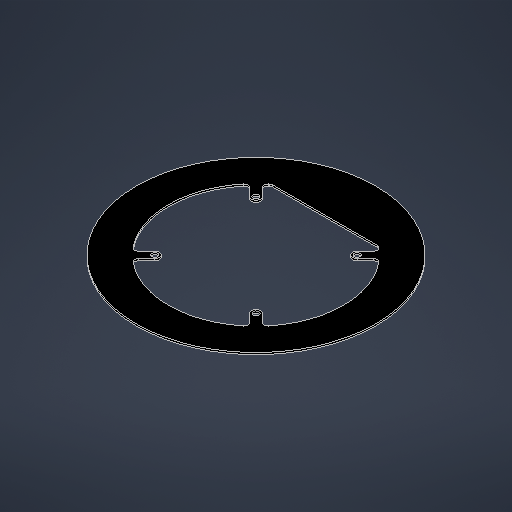
# Autodesk Inventor part: InfraredPCB
Saved by Autodesk Inventor 2025.2 (Build 292293000, 293)
## iProperties
Created: 2023-03-06
Part Number: InfraredPCB
Material: Generic
Document SubType Name: Modeling
Designer: Elias Braun
Density: 1 g/cm^3
Appearance: Default
Author: Elias Braun
Autodesk Inventor part; units mm, degrees
ref_plane "YZ Plane" through (0, 0, 0) normal (1, 0, 0) x (0, 1, 0)
ref_plane "XZ Plane" through (0, 0, 0) normal (0, 1, 0) x (-1, 0, 0)
ref_plane "XY Plane" through (0, 0, 0) normal (0, 0, 1) x (1, 0, 0)
sketch "Sketch3" plane through (0, 0, 0) normal (0, 1, 0) x (-1, 0, 0)
  line L0 (27.5, -27.5) -> (-27.5, -27.5) construction
  line L1 (-27.5, -27.5) -> (-27.5, 27.5) construction
  line L2 (-27.5, 27.5) -> (27.5, 27.5) construction
  line L3 (27.5, 27.5) -> (27.5, -27.5) construction
  line L4 (27.5, -27.5) -> (-27.5, 27.5) construction
  line L5 (-27.5, -27.5) -> (27.5, 27.5) construction
  circle A0 centre (27.5, -27.5) radius 1.6
  circle A1 centre (-27.5, -27.5) radius 1.6
  circle A2 centre (-27.5, 27.5) radius 1.6
  circle A3 centre (27.5, 27.5) radius 1.6
  circle A4 centre (0, 0) radius 65
  line L6 (-27.5, -27.5) -> (-33.5876, -33.5876) construction
  line L7 (-27.5, 27.5) -> (-33.5876, 33.5876) construction
  line L8 (27.5, 27.5) -> (33.5876, 33.5876) construction
  line L9 (27.5, -27.5) -> (33.5876, -33.5876) construction
  line L10 (39.6751, -39.6751) -> (27.5, -27.5) construction
  line L11 (35.3088, -31.7733) -> (29.2678, -25.7322)
  line L12 (25.7322, -29.2678) -> (31.7733, -35.3088)
  arc A5 (29.2678, -25.7322) -> (25.7322, -29.2678) centre (27.5, -27.5) ccw
  line L13 (-39.6751, -39.6751) -> (-27.5, -27.5) construction
  line L14 (-31.7733, -35.3088) -> (-25.7322, -29.2678)
  line L15 (-29.2678, -25.7322) -> (-35.3088, -31.7733)
  arc A6 (-25.7322, -29.2678) -> (-29.2678, -25.7322) centre (-27.5, -27.5) ccw
  line L16 (-39.6751, 39.6751) -> (-27.5, 27.5) construction
  line L17 (-35.3088, 31.7733) -> (-29.2678, 25.7322)
  line L18 (-25.7322, 29.2678) -> (-31.7733, 35.3088)
  arc A7 (-29.2678, 25.7322) -> (-25.7322, 29.2678) centre (-27.5, 27.5) ccw
  line L19 (33.5876, 33.5876) -> (27.5, 27.5) construction
  line L20 (31.7733, 35.3088) -> (25.7322, 29.2678)
  line L21 (29.2678, 25.7322) -> (35.3088, 31.7733)
  arc A8 (25.7322, 29.2678) -> (29.2678, 25.7322) centre (27.5, 27.5) ccw
  arc A9 (31.7733, 35.3088) -> (-31.7733, 35.3088) centre (0, 0) ccw
  arc A10 (-35.3088, 31.7733) -> (-35.3088, -31.7733) centre (0, 0) ccw
  arc A11 (-31.7733, -35.3088) -> (31.7733, -35.3088) centre (0, 0) ccw
  arc A12 (35.3088, -31.7733) -> (35.3088, 31.7733) centre (0, 0) ccw
  line L22 (0, -47.5) -> (0, -37.5) construction
  line L23 (0, -37.5) -> (-29.1548, -37.5)
  line L24 (0, -37.5) -> (29.1548, -37.5)
  dimension "d60" = 55
  dimension "d61" = 55
  dimension "d62" = 3.2
  dimension "d63" = 3.2
  dimension "d64" = 3.2
  dimension "d65" = 3.2
  dimension "d67" = 130
  dimension "d68" = 5
  dimension "d69" = 5
  dimension "d70" = 5
  dimension "d71" = 5
  dimension "d91" = 10
  constraints: 58 end point, 21 point on circle, 13 centre point, 8 tangent, 6 coincident, 6 parallel, 5 midpoint, 4 collinear, 4 point on line, 3 perpendicular, 1 horizontal, 1 vertical
  measures "d60" distance of L0.start L0.end
  measures "d61" distance of L0.end L1.end
  measures "d62" diameter of A0
  measures "d63" diameter of A1
  measures "d64" diameter of A2
  measures "d65" diameter of A3
  measures "d67" diameter of A4
  measures "d68" diameter of A5
  measures "d69" diameter of A6
  measures "d70" diameter of A7
  measures "d71" diameter of A8
  measures "d91" distance of L22.start L22.end
extrude "Extrusion2" add sketch "Sketch3" along normal blind 1 contours A4 | A11 L23 L24
fillet "Fillet1" radius 2 10 edges at (-31.7733, 0.5, 35.3088) (-35.3088, 0.5, 31.7733) (-31.7733, 0.5, -35.3088) (-35.3088, 0.5, -31.7733) (35.3088, 0.5, -31.7733) (31.7733, 0.5, -35.3088) (31.7733, 0.5, 35.3088) (35.3088, 0.5, 31.7733) (-29.1548, 0.5, -37.5) (29.1548, 0.5, -37.5)
sketch "Sketch4" plane through (0, 1, 0) normal (0, 1, 0) x (1, 0, 0)
  circle A0 centre (0, 0) radius 65 projected
  line L0 (0, -65) -> (0, -63) construction
  line L1 (-3, -57) -> (-3, -63)
  line L2 (-3, -63) -> (3, -63)
  line L3 (3, -63) -> (3, -57)
  line L4 (3, -57) -> (-3, -57)
  line L5 (0.8, -52.3) -> (0.8, -55.5)
  line L6 (0.8, -55.5) -> (-0.8, -55.5)
  line L7 (-0.8, -55.5) -> (-0.8, -52.3)
  line L8 (-0.8, -52.3) -> (0.8, -52.3)
  line L9 (1.8, -52.3) -> (1.8, -55.5)
  line L10 (1.8, -55.5) -> (3.4, -55.5)
  line L11 (3.4, -55.5) -> (3.4, -52.3)
  line L12 (3.4, -52.3) -> (1.8, -52.3)
  line L13 (-3.4, -52.3) -> (-3.4, -55.5)
  line L14 (-3.4, -55.5) -> (-1.8, -55.5)
  line L15 (-1.8, -55.5) -> (-1.8, -52.3)
  line L16 (-1.8, -52.3) -> (-3.4, -52.3)
  line L17 (-4.4, -52.3) -> (-4.4, -55.5)
  line L18 (-4.4, -55.5) -> (-6, -55.5)
  line L19 (-6, -55.5) -> (-6, -52.3)
  line L20 (-6, -52.3) -> (-4.4, -52.3)
  line L21 (-4.4, -61.6) -> (-4.4, -58.4)
  line L22 (-4.4, -58.4) -> (-6, -58.4)
  line L23 (-6, -58.4) -> (-6, -61.6)
  line L24 (-6, -61.6) -> (-4.4, -61.6)
  line L25 (18.0977, -52.5764) -> (19.5759, -51.9641)
  line L26 (19.5759, -51.9641) -> (18.3514, -49.0077)
  line L27 (18.3514, -49.0077) -> (16.8732, -49.62)
  line L28 (16.8732, -49.62) -> (18.0977, -52.5764)
  line L29 (15.9493, -50.0027) -> (17.1739, -52.9591)
  line L30 (15.6957, -53.5714) -> (14.4711, -50.615)
  line L31 (14.4711, -50.615) -> (15.9493, -50.0027)
  line L32 (17.1739, -52.9591) -> (15.6957, -53.5714)
  line L33 (18.2836, -55.6384) -> (16.8054, -56.2507)
  line L34 (16.8054, -56.2507) -> (18.03, -59.2071)
  line L35 (18.03, -59.2071) -> (19.5082, -58.5948)
  line L36 (19.5082, -58.5948) -> (18.2836, -55.6384)
  line L37 (19.0413, -53.8092) -> (21.3374, -59.3525)
  line L38 (21.3374, -59.3525) -> (26.8807, -57.0564)
  line L39 (24.8744, -60.0522) -> (24.1091, -58.2044) construction
  line L40 (26.8807, -57.0564) -> (24.5846, -51.5131)
  line L41 (24.5846, -51.5131) -> (19.0413, -53.8092)
  line L42 (20.7534, -48.0128) -> (21.978, -50.9692)
  line L43 (21.978, -50.9692) -> (20.4998, -51.5815)
  line L44 (20.4998, -51.5815) -> (19.2752, -48.625)
  line L45 (19.2752, -48.625) -> (20.7534, -48.0128)
  line L46 (21.6773, -47.6301) -> (22.9019, -50.5865)
  line L47 (22.9019, -50.5865) -> (24.3801, -49.9742)
  line L48 (24.3801, -49.9742) -> (23.1555, -47.0178)
  line L49 (23.1555, -47.0178) -> (21.6773, -47.6301)
  line L50 (36.8403, -41.6486) -> (37.9716, -40.5172)
  line L51 (37.9716, -40.5172) -> (35.7089, -38.2545)
  line L52 (35.7089, -38.2545) -> (34.5775, -39.3858)
  line L53 (34.5775, -39.3858) -> (36.8403, -41.6486)
  line L54 (33.8704, -40.093) -> (36.1332, -42.3557)
  line L55 (35.0018, -43.4871) -> (32.739, -41.2243)
  line L56 (32.739, -41.2243) -> (33.8704, -40.093)
  line L57 (36.1332, -42.3557) -> (35.0018, -43.4871)
  line L58 (38.1838, -44.4063) -> (37.0524, -45.5377)
  line L59 (37.0524, -45.5377) -> (39.3151, -47.8004)
  line L60 (39.3151, -47.8004) -> (40.4465, -46.669)
  line L61 (40.4465, -46.669) -> (38.1838, -44.4063)
  line L62 (38.1838, -42.4264) -> (42.4264, -46.669)
  line L63 (42.4264, -46.669) -> (46.669, -42.4264)
  line L64 (45.9619, -45.9619) -> (44.5477, -44.5477) construction
  line L65 (46.669, -42.4264) -> (42.4264, -38.1838)
  line L66 (42.4264, -38.1838) -> (38.1838, -42.4264)
  line L67 (37.5474, -36.416) -> (39.8101, -38.6787)
  line L68 (39.8101, -38.6787) -> (38.6787, -39.8101)
  line L69 (38.6787, -39.8101) -> (36.416, -37.5474)
  line L70 (36.416, -37.5474) -> (37.5474, -36.416)
  line L71 (38.2545, -35.7089) -> (40.5172, -37.9716)
  line L72 (40.5172, -37.9716) -> (41.6486, -36.8403)
  line L73 (41.6486, -36.8403) -> (39.3858, -34.5775)
  line L74 (39.3858, -34.5775) -> (38.2545, -35.7089)
  line L75 (49.9742, -24.3801) -> (50.5865, -22.9019)
  line L76 (50.5865, -22.9019) -> (47.6301, -21.6773)
  line L77 (47.6301, -21.6773) -> (47.0178, -23.1555)
  line L78 (47.0178, -23.1555) -> (49.9742, -24.3801)
  line L79 (46.6351, -24.0794) -> (49.5915, -25.304)
  line L80 (48.9792, -26.7822) -> (46.0228, -25.5576)
  line L81 (46.0228, -25.5576) -> (46.6351, -24.0794)
  line L82 (49.5915, -25.304) -> (48.9792, -26.7822)
  line L83 (52.2708, -26.4138) -> (51.6585, -27.892)
  line L84 (51.6585, -27.892) -> (54.6149, -29.1166)
  line L85 (54.6149, -29.1166) -> (55.2272, -27.6384)
  line L86 (55.2272, -27.6384) -> (52.2708, -26.4138)
  line L87 (51.5131, -24.5846) -> (57.0564, -26.8807)
  line L88 (57.0564, -26.8807) -> (59.3525, -21.3374)
  line L89 (60.0522, -24.8744) -> (58.2044, -24.1091) construction
  line L90 (59.3525, -21.3374) -> (53.8092, -19.0413)
  line L91 (53.8092, -19.0413) -> (51.5131, -24.5846)
  line L92 (48.625, -19.2752) -> (51.5815, -20.4998)
  line L93 (51.5815, -20.4998) -> (50.9692, -21.978)
  line L94 (50.9692, -21.978) -> (48.0128, -20.7534)
  line L95 (48.0128, -20.7534) -> (48.625, -19.2752)
  line L96 (49.0077, -18.3514) -> (51.9641, -19.5759)
  line L97 (51.9641, -19.5759) -> (52.5764, -18.0977)
  line L98 (52.5764, -18.0977) -> (49.62, -16.8732)
  line L99 (49.62, -16.8732) -> (49.0077, -18.3514)
  line L100 (55.5, -3.4) -> (55.5, -1.8)
  line L101 (55.5, -1.8) -> (52.3, -1.8)
  line L102 (52.3, -1.8) -> (52.3, -3.4)
  line L103 (52.3, -3.4) -> (55.5, -3.4)
  line L104 (52.3, -4.4) -> (55.5, -4.4)
  line L105 (55.5, -6) -> (52.3, -6)
  line L106 (52.3, -6) -> (52.3, -4.4)
  line L107 (55.5, -4.4) -> (55.5, -6)
  line L108 (58.4, -4.4) -> (58.4, -6)
  line L109 (58.4, -6) -> (61.6, -6)
  line L110 (61.6, -6) -> (61.6, -4.4)
  line L111 (61.6, -4.4) -> (58.4, -4.4)
  line L112 (57, -3) -> (63, -3)
  line L113 (63, -3) -> (63, 3)
  line L114 (65, 0) -> (63, 0) construction
  line L115 (63, 3) -> (57, 3)
  line L116 (57, 3) -> (57, -3)
  line L117 (52.3, 0.8) -> (55.5, 0.8)
  line L118 (55.5, 0.8) -> (55.5, -0.8)
  line L119 (55.5, -0.8) -> (52.3, -0.8)
  line L120 (52.3, -0.8) -> (52.3, 0.8)
  line L121 (52.3, 1.8) -> (55.5, 1.8)
  line L122 (55.5, 1.8) -> (55.5, 3.4)
  line L123 (55.5, 3.4) -> (52.3, 3.4)
  line L124 (52.3, 3.4) -> (52.3, 1.8)
  line L125 (52.5764, 18.0977) -> (51.9641, 19.5759)
  line L126 (51.9641, 19.5759) -> (49.0077, 18.3514)
  line L127 (49.0077, 18.3514) -> (49.62, 16.8732)
  line L128 (49.62, 16.8732) -> (52.5764, 18.0977)
  line L129 (50.0027, 15.9493) -> (52.9591, 17.1739)
  line L130 (53.5714, 15.6957) -> (50.615, 14.4711)
  line L131 (50.615, 14.4711) -> (50.0027, 15.9493)
  line L132 (52.9591, 17.1739) -> (53.5714, 15.6957)
  line L133 (55.6384, 18.2836) -> (56.2507, 16.8054)
  line L134 (56.2507, 16.8054) -> (59.2071, 18.03)
  line L135 (59.2071, 18.03) -> (58.5948, 19.5082)
  line L136 (58.5948, 19.5082) -> (55.6384, 18.2836)
  line L137 (53.8092, 19.0413) -> (59.3525, 21.3374)
  line L138 (59.3525, 21.3374) -> (57.0564, 26.8807)
  line L139 (60.0522, 24.8744) -> (58.2044, 24.1091) construction
  line L140 (57.0564, 26.8807) -> (51.5131, 24.5846)
  line L141 (51.5131, 24.5846) -> (53.8092, 19.0413)
  line L142 (48.0128, 20.7534) -> (50.9692, 21.978)
  line L143 (50.9692, 21.978) -> (51.5815, 20.4998)
  line L144 (51.5815, 20.4998) -> (48.625, 19.2752)
  line L145 (48.625, 19.2752) -> (48.0128, 20.7534)
  line L146 (47.6301, 21.6773) -> (50.5865, 22.9019)
  line L147 (50.5865, 22.9019) -> (49.9742, 24.3801)
  line L148 (49.9742, 24.3801) -> (47.0178, 23.1555)
  line L149 (47.0178, 23.1555) -> (47.6301, 21.6773)
  line L150 (41.6486, 36.8403) -> (40.5172, 37.9716)
  line L151 (40.5172, 37.9716) -> (38.2545, 35.7089)
  line L152 (38.2545, 35.7089) -> (39.3858, 34.5775)
  line L153 (39.3858, 34.5775) -> (41.6486, 36.8403)
  line L154 (40.093, 33.8704) -> (42.3557, 36.1332)
  line L155 (43.4871, 35.0018) -> (41.2243, 32.739)
  line L156 (41.2243, 32.739) -> (40.093, 33.8704)
  line L157 (42.3557, 36.1332) -> (43.4871, 35.0018)
  line L158 (44.4063, 38.1838) -> (45.5377, 37.0524)
  line L159 (45.5377, 37.0524) -> (47.8004, 39.3151)
  line L160 (47.8004, 39.3151) -> (46.669, 40.4465)
  line L161 (46.669, 40.4465) -> (44.4063, 38.1838)
  line L162 (42.4264, 38.1838) -> (46.669, 42.4264)
  line L163 (46.669, 42.4264) -> (42.4264, 46.669)
  line L164 (45.9619, 45.9619) -> (44.5477, 44.5477) construction
  line L165 (42.4264, 46.669) -> (38.1838, 42.4264)
  line L166 (38.1838, 42.4264) -> (42.4264, 38.1838)
  line L167 (36.416, 37.5474) -> (38.6787, 39.8101)
  line L168 (38.6787, 39.8101) -> (39.8101, 38.6787)
  line L169 (39.8101, 38.6787) -> (37.5474, 36.416)
  line L170 (37.5474, 36.416) -> (36.416, 37.5474)
  line L171 (35.7089, 38.2545) -> (37.9716, 40.5172)
  line L172 (37.9716, 40.5172) -> (36.8403, 41.6486)
  line L173 (36.8403, 41.6486) -> (34.5775, 39.3858)
  line L174 (34.5775, 39.3858) -> (35.7089, 38.2545)
  line L175 (24.3801, 49.9742) -> (22.9019, 50.5865)
  line L176 (22.9019, 50.5865) -> (21.6773, 47.6301)
  line L177 (21.6773, 47.6301) -> (23.1555, 47.0178)
  line L178 (23.1555, 47.0178) -> (24.3801, 49.9742)
  line L179 (24.0794, 46.6351) -> (25.304, 49.5915)
  line L180 (26.7822, 48.9792) -> (25.5576, 46.0228)
  line L181 (25.5576, 46.0228) -> (24.0794, 46.6351)
  line L182 (25.304, 49.5915) -> (26.7822, 48.9792)
  line L183 (26.4138, 52.2708) -> (27.892, 51.6585)
  line L184 (27.892, 51.6585) -> (29.1166, 54.6149)
  line L185 (29.1166, 54.6149) -> (27.6384, 55.2272)
  line L186 (27.6384, 55.2272) -> (26.4138, 52.2708)
  line L187 (24.5846, 51.5131) -> (26.8807, 57.0564)
  line L188 (26.8807, 57.0564) -> (21.3374, 59.3525)
  line L189 (24.8744, 60.0522) -> (24.1091, 58.2044) construction
  line L190 (21.3374, 59.3525) -> (19.0413, 53.8092)
  line L191 (19.0413, 53.8092) -> (24.5846, 51.5131)
  line L192 (19.2752, 48.625) -> (20.4998, 51.5815)
  line L193 (20.4998, 51.5815) -> (21.978, 50.9692)
  line L194 (21.978, 50.9692) -> (20.7534, 48.0128)
  line L195 (20.7534, 48.0128) -> (19.2752, 48.625)
  line L196 (18.3514, 49.0077) -> (19.5759, 51.9641)
  line L197 (19.5759, 51.9641) -> (18.0977, 52.5764)
  line L198 (18.0977, 52.5764) -> (16.8732, 49.62)
  line L199 (16.8732, 49.62) -> (18.3514, 49.0077)
  line L200 (3.4, 55.5) -> (1.8, 55.5)
  line L201 (1.8, 55.5) -> (1.8, 52.3)
  line L202 (1.8, 52.3) -> (3.4, 52.3)
  line L203 (3.4, 52.3) -> (3.4, 55.5)
  line L204 (4.4, 52.3) -> (4.4, 55.5)
  line L205 (6, 55.5) -> (6, 52.3)
  line L206 (6, 52.3) -> (4.4, 52.3)
  line L207 (4.4, 55.5) -> (6, 55.5)
  line L208 (4.4, 58.4) -> (6, 58.4)
  line L209 (6, 58.4) -> (6, 61.6)
  line L210 (6, 61.6) -> (4.4, 61.6)
  line L211 (4.4, 61.6) -> (4.4, 58.4)
  line L212 (3, 57) -> (3, 63)
  line L213 (3, 63) -> (-3, 63)
  line L214 (0, 65) -> (0, 63) construction
  line L215 (-3, 63) -> (-3, 57)
  line L216 (-3, 57) -> (3, 57)
  line L217 (-0.8, 52.3) -> (-0.8, 55.5)
  line L218 (-0.8, 55.5) -> (0.8, 55.5)
  line L219 (0.8, 55.5) -> (0.8, 52.3)
  line L220 (0.8, 52.3) -> (-0.8, 52.3)
  line L221 (-1.8, 52.3) -> (-1.8, 55.5)
  line L222 (-1.8, 55.5) -> (-3.4, 55.5)
  line L223 (-3.4, 55.5) -> (-3.4, 52.3)
  line L224 (-3.4, 52.3) -> (-1.8, 52.3)
  line L225 (-18.0977, 52.5764) -> (-19.5759, 51.9641)
  line L226 (-19.5759, 51.9641) -> (-18.3514, 49.0077)
  line L227 (-18.3514, 49.0077) -> (-16.8732, 49.62)
  line L228 (-16.8732, 49.62) -> (-18.0977, 52.5764)
  line L229 (-15.9493, 50.0027) -> (-17.1739, 52.9591)
  line L230 (-15.6957, 53.5714) -> (-14.4711, 50.615)
  line L231 (-14.4711, 50.615) -> (-15.9493, 50.0027)
  line L232 (-17.1739, 52.9591) -> (-15.6957, 53.5714)
  line L233 (-18.2836, 55.6384) -> (-16.8054, 56.2507)
  line L234 (-16.8054, 56.2507) -> (-18.03, 59.2071)
  line L235 (-18.03, 59.2071) -> (-19.5082, 58.5948)
  line L236 (-19.5082, 58.5948) -> (-18.2836, 55.6384)
  line L237 (-19.0413, 53.8092) -> (-21.3374, 59.3525)
  line L238 (-21.3374, 59.3525) -> (-26.8807, 57.0564)
  line L239 (-24.8744, 60.0522) -> (-24.1091, 58.2044) construction
  line L240 (-26.8807, 57.0564) -> (-24.5846, 51.5131)
  line L241 (-24.5846, 51.5131) -> (-19.0413, 53.8092)
  line L242 (-20.7534, 48.0128) -> (-21.978, 50.9692)
  line L243 (-21.978, 50.9692) -> (-20.4998, 51.5815)
  line L244 (-20.4998, 51.5815) -> (-19.2752, 48.625)
  line L245 (-19.2752, 48.625) -> (-20.7534, 48.0128)
  line L246 (-21.6773, 47.6301) -> (-22.9019, 50.5865)
  line L247 (-22.9019, 50.5865) -> (-24.3801, 49.9742)
  line L248 (-24.3801, 49.9742) -> (-23.1555, 47.0178)
  line L249 (-23.1555, 47.0178) -> (-21.6773, 47.6301)
  line L250 (-36.8403, 41.6486) -> (-37.9716, 40.5172)
  line L251 (-37.9716, 40.5172) -> (-35.7089, 38.2545)
  line L252 (-35.7089, 38.2545) -> (-34.5775, 39.3858)
  line L253 (-34.5775, 39.3858) -> (-36.8403, 41.6486)
  line L254 (-33.8704, 40.093) -> (-36.1332, 42.3557)
  line L255 (-35.0018, 43.4871) -> (-32.739, 41.2243)
  line L256 (-32.739, 41.2243) -> (-33.8704, 40.093)
  line L257 (-36.1332, 42.3557) -> (-35.0018, 43.4871)
  line L258 (-38.1838, 44.4063) -> (-37.0524, 45.5377)
  line L259 (-37.0524, 45.5377) -> (-39.3151, 47.8004)
  line L260 (-39.3151, 47.8004) -> (-40.4465, 46.669)
  line L261 (-40.4465, 46.669) -> (-38.1838, 44.4063)
  line L262 (-38.1838, 42.4264) -> (-42.4264, 46.669)
  line L263 (-42.4264, 46.669) -> (-46.669, 42.4264)
  line L264 (-45.9619, 45.9619) -> (-44.5477, 44.5477) construction
  line L265 (-46.669, 42.4264) -> (-42.4264, 38.1838)
  line L266 (-42.4264, 38.1838) -> (-38.1838, 42.4264)
  line L267 (-37.5474, 36.416) -> (-39.8101, 38.6787)
  line L268 (-39.8101, 38.6787) -> (-38.6787, 39.8101)
  line L269 (-38.6787, 39.8101) -> (-36.416, 37.5474)
  line L270 (-36.416, 37.5474) -> (-37.5474, 36.416)
  line L271 (-38.2545, 35.7089) -> (-40.5172, 37.9716)
  line L272 (-40.5172, 37.9716) -> (-41.6486, 36.8403)
  line L273 (-41.6486, 36.8403) -> (-39.3858, 34.5775)
  line L274 (-39.3858, 34.5775) -> (-38.2545, 35.7089)
  line L275 (-49.9742, 24.3801) -> (-50.5865, 22.9019)
  line L276 (-50.5865, 22.9019) -> (-47.6301, 21.6773)
  line L277 (-47.6301, 21.6773) -> (-47.0178, 23.1555)
  line L278 (-47.0178, 23.1555) -> (-49.9742, 24.3801)
  line L279 (-46.6351, 24.0794) -> (-49.5915, 25.304)
  line L280 (-48.9792, 26.7822) -> (-46.0228, 25.5576)
  line L281 (-46.0228, 25.5576) -> (-46.6351, 24.0794)
  line L282 (-49.5915, 25.304) -> (-48.9792, 26.7822)
  line L283 (-52.2708, 26.4138) -> (-51.6585, 27.892)
  line L284 (-51.6585, 27.892) -> (-54.6149, 29.1166)
  line L285 (-54.6149, 29.1166) -> (-55.2272, 27.6384)
  line L286 (-55.2272, 27.6384) -> (-52.2708, 26.4138)
  line L287 (-51.5131, 24.5846) -> (-57.0564, 26.8807)
  line L288 (-57.0564, 26.8807) -> (-59.3525, 21.3374)
  line L289 (-60.0522, 24.8744) -> (-58.2044, 24.1091) construction
  line L290 (-59.3525, 21.3374) -> (-53.8092, 19.0413)
  line L291 (-53.8092, 19.0413) -> (-51.5131, 24.5846)
  line L292 (-48.625, 19.2752) -> (-51.5815, 20.4998)
  line L293 (-51.5815, 20.4998) -> (-50.9692, 21.978)
  line L294 (-50.9692, 21.978) -> (-48.0128, 20.7534)
  line L295 (-48.0128, 20.7534) -> (-48.625, 19.2752)
  line L296 (-49.0077, 18.3514) -> (-51.9641, 19.5759)
  line L297 (-51.9641, 19.5759) -> (-52.5764, 18.0977)
  line L298 (-52.5764, 18.0977) -> (-49.62, 16.8732)
  line L299 (-49.62, 16.8732) -> (-49.0077, 18.3514)
  line L300 (-55.5, 3.4) -> (-55.5, 1.8)
  line L301 (-55.5, 1.8) -> (-52.3, 1.8)
  line L302 (-52.3, 1.8) -> (-52.3, 3.4)
  line L303 (-52.3, 3.4) -> (-55.5, 3.4)
  line L304 (-52.3, 4.4) -> (-55.5, 4.4)
  line L305 (-55.5, 6) -> (-52.3, 6)
  line L306 (-52.3, 6) -> (-52.3, 4.4)
  line L307 (-55.5, 4.4) -> (-55.5, 6)
  line L308 (-58.4, 4.4) -> (-58.4, 6)
  line L309 (-58.4, 6) -> (-61.6, 6)
  line L310 (-61.6, 6) -> (-61.6, 4.4)
  line L311 (-61.6, 4.4) -> (-58.4, 4.4)
  line L312 (-57, 3) -> (-63, 3)
  line L313 (-63, 3) -> (-63, -3)
  line L314 (-65, 0) -> (-63, 0) construction
  line L315 (-63, -3) -> (-57, -3)
  line L316 (-57, -3) -> (-57, 3)
  line L317 (-52.3, -0.8) -> (-55.5, -0.8)
  line L318 (-55.5, -0.8) -> (-55.5, 0.8)
  line L319 (-55.5, 0.8) -> (-52.3, 0.8)
  line L320 (-52.3, 0.8) -> (-52.3, -0.8)
  line L321 (-52.3, -1.8) -> (-55.5, -1.8)
  line L322 (-55.5, -1.8) -> (-55.5, -3.4)
  line L323 (-55.5, -3.4) -> (-52.3, -3.4)
  line L324 (-52.3, -3.4) -> (-52.3, -1.8)
  line L325 (-52.5764, -18.0977) -> (-51.9641, -19.5759)
  line L326 (-51.9641, -19.5759) -> (-49.0077, -18.3514)
  line L327 (-49.0077, -18.3514) -> (-49.62, -16.8732)
  line L328 (-49.62, -16.8732) -> (-52.5764, -18.0977)
  line L329 (-50.0027, -15.9493) -> (-52.9591, -17.1739)
  line L330 (-53.5714, -15.6957) -> (-50.615, -14.4711)
  line L331 (-50.615, -14.4711) -> (-50.0027, -15.9493)
  line L332 (-52.9591, -17.1739) -> (-53.5714, -15.6957)
  line L333 (-55.6384, -18.2836) -> (-56.2507, -16.8054)
  line L334 (-56.2507, -16.8054) -> (-59.2071, -18.03)
  line L335 (-59.2071, -18.03) -> (-58.5948, -19.5082)
  line L336 (-58.5948, -19.5082) -> (-55.6384, -18.2836)
  line L337 (-53.8092, -19.0413) -> (-59.3525, -21.3374)
  line L338 (-59.3525, -21.3374) -> (-57.0564, -26.8807)
  line L339 (-60.0522, -24.8744) -> (-58.2044, -24.1091) construction
  line L340 (-57.0564, -26.8807) -> (-51.5131, -24.5846)
  line L341 (-51.5131, -24.5846) -> (-53.8092, -19.0413)
  line L342 (-48.0128, -20.7534) -> (-50.9692, -21.978)
  line L343 (-50.9692, -21.978) -> (-51.5815, -20.4998)
  line L344 (-51.5815, -20.4998) -> (-48.625, -19.2752)
  line L345 (-48.625, -19.2752) -> (-48.0128, -20.7534)
  line L346 (-47.6301, -21.6773) -> (-50.5865, -22.9019)
  line L347 (-50.5865, -22.9019) -> (-49.9742, -24.3801)
  line L348 (-49.9742, -24.3801) -> (-47.0178, -23.1555)
  line L349 (-47.0178, -23.1555) -> (-47.6301, -21.6773)
  line L350 (-41.6486, -36.8403) -> (-40.5172, -37.9716)
  line L351 (-40.5172, -37.9716) -> (-38.2545, -35.7089)
  line L352 (-38.2545, -35.7089) -> (-39.3858, -34.5775)
  line L353 (-39.3858, -34.5775) -> (-41.6486, -36.8403)
  line L354 (-40.093, -33.8704) -> (-42.3557, -36.1332)
  line L355 (-43.4871, -35.0018) -> (-41.2243, -32.739)
  line L356 (-41.2243, -32.739) -> (-40.093, -33.8704)
  line L357 (-42.3557, -36.1332) -> (-43.4871, -35.0018)
  line L358 (-44.4063, -38.1838) -> (-45.5377, -37.0524)
  line L359 (-45.5377, -37.0524) -> (-47.8004, -39.3151)
  line L360 (-47.8004, -39.3151) -> (-46.669, -40.4465)
  line L361 (-46.669, -40.4465) -> (-44.4063, -38.1838)
  line L362 (-42.4264, -38.1838) -> (-46.669, -42.4264)
  line L363 (-46.669, -42.4264) -> (-42.4264, -46.669)
  line L364 (-45.9619, -45.9619) -> (-44.5477, -44.5477) construction
  line L365 (-42.4264, -46.669) -> (-38.1838, -42.4264)
  line L366 (-38.1838, -42.4264) -> (-42.4264, -38.1838)
  line L367 (-36.416, -37.5474) -> (-38.6787, -39.8101)
  line L368 (-38.6787, -39.8101) -> (-39.8101, -38.6787)
  line L369 (-39.8101, -38.6787) -> (-37.5474, -36.416)
  line L370 (-37.5474, -36.416) -> (-36.416, -37.5474)
  line L371 (-35.7089, -38.2545) -> (-37.9716, -40.5172)
  line L372 (-37.9716, -40.5172) -> (-36.8403, -41.6486)
  line L373 (-36.8403, -41.6486) -> (-34.5775, -39.3858)
  line L374 (-34.5775, -39.3858) -> (-35.7089, -38.2545)
  line L375 (-24.3801, -49.9742) -> (-22.9019, -50.5865)
  line L376 (-22.9019, -50.5865) -> (-21.6773, -47.6301)
  line L377 (-21.6773, -47.6301) -> (-23.1555, -47.0178)
  line L378 (-23.1555, -47.0178) -> (-24.3801, -49.9742)
  line L379 (-24.0794, -46.6351) -> (-25.304, -49.5915)
  line L380 (-26.7822, -48.9792) -> (-25.5576, -46.0228)
  line L381 (-25.5576, -46.0228) -> (-24.0794, -46.6351)
  line L382 (-25.304, -49.5915) -> (-26.7822, -48.9792)
  line L383 (-26.4138, -52.2708) -> (-27.892, -51.6585)
  line L384 (-27.892, -51.6585) -> (-29.1166, -54.6149)
  line L385 (-29.1166, -54.6149) -> (-27.6384, -55.2272)
  line L386 (-27.6384, -55.2272) -> (-26.4138, -52.2708)
  line L387 (-24.5846, -51.5131) -> (-26.8807, -57.0564)
  line L388 (-26.8807, -57.0564) -> (-21.3374, -59.3525)
  line L389 (-24.8744, -60.0522) -> (-24.1091, -58.2044) construction
  line L390 (-21.3374, -59.3525) -> (-19.0413, -53.8092)
  line L391 (-19.0413, -53.8092) -> (-24.5846, -51.5131)
  line L392 (-19.2752, -48.625) -> (-20.4998, -51.5815)
  line L393 (-20.4998, -51.5815) -> (-21.978, -50.9692)
  line L394 (-21.978, -50.9692) -> (-20.7534, -48.0128)
  line L395 (-20.7534, -48.0128) -> (-19.2752, -48.625)
  line L396 (-18.3514, -49.0077) -> (-19.5759, -51.9641)
  line L397 (-19.5759, -51.9641) -> (-18.0977, -52.5764)
  line L398 (-18.0977, -52.5764) -> (-16.8732, -49.62)
  line L399 (-16.8732, -49.62) -> (-18.3514, -49.0077)
  point P0 (0, -53.9)
  point P1 (0, -60)
  point P2 (2.6, -53.9)
  point P3 (-2.6, -53.9)
  point P4 (-5.2, -53.9)
  point P5 (-5.2, -60)
  point P6 (18.1568, -57.4227)
  point P7 (15.8225, -51.7871)
  point P8 (18.2246, -50.7921)
  point P9 (23.0287, -48.8021)
  point P10 (22.961, -55.4328)
  point P11 (20.6266, -49.7971)
  point P12 (38.7495, -46.1034)
  point P13 (34.4361, -41.79)
  point P14 (36.2746, -39.9515)
  point P15 (39.9515, -36.2746)
  point P16 (42.4264, -42.4264)
  point P17 (38.1131, -38.1131)
  point P18 (53.4428, -27.7652)
  point P19 (47.8072, -25.4308)
  point P20 (48.8021, -23.0287)
  point P21 (50.7921, -18.2246)
  point P22 (55.4328, -22.961)
  point P23 (49.7971, -20.6266)
  point P24 (60, -5.2)
  point P25 (53.9, -5.2)
  point P26 (53.9, -2.6)
  point P27 (53.9, 2.6)
  point P28 (60, 0)
  point P29 (53.9, 0)
  point P30 (57.4227, 18.1568)
  point P31 (51.7871, 15.8225)
  point P32 (50.7921, 18.2246)
  point P33 (48.8021, 23.0287)
  point P34 (55.4328, 22.961)
  point P35 (49.7971, 20.6266)
  point P36 (46.1034, 38.7495)
  point P37 (41.79, 34.4361)
  point P38 (39.9515, 36.2746)
  point P39 (36.2746, 39.9515)
  point P40 (42.4264, 42.4264)
  point P41 (38.1131, 38.1131)
  point P42 (27.7652, 53.4428)
  point P43 (25.4308, 47.8072)
  point P44 (23.0287, 48.8021)
  point P45 (18.2246, 50.7921)
  point P46 (22.961, 55.4328)
  point P47 (20.6266, 49.7971)
  point P48 (5.2, 60)
  point P49 (5.2, 53.9)
  point P50 (2.6, 53.9)
  point P51 (-2.6, 53.9)
  point P52 (0, 60)
  point P53 (0, 53.9)
  point P54 (-18.1568, 57.4227)
  point P55 (-15.8225, 51.7871)
  point P56 (-18.2246, 50.7921)
  point P57 (-23.0287, 48.8021)
  point P58 (-22.961, 55.4328)
  point P59 (-20.6266, 49.7971)
  point P60 (-38.7495, 46.1034)
  point P61 (-34.4361, 41.79)
  point P62 (-36.2746, 39.9515)
  point P63 (-39.9515, 36.2746)
  point P64 (-42.4264, 42.4264)
  point P65 (-38.1131, 38.1131)
  point P66 (-53.4428, 27.7652)
  point P67 (-47.8072, 25.4308)
  point P68 (-48.8021, 23.0287)
  point P69 (-50.7921, 18.2246)
  point P70 (-55.4328, 22.961)
  point P71 (-49.7971, 20.6266)
  point P72 (-60, 5.2)
  point P73 (-53.9, 5.2)
  point P74 (-53.9, 2.6)
  point P75 (-53.9, -2.6)
  point P76 (-60, 0)
  point P77 (-53.9, 0)
  point P78 (-57.4227, -18.1568)
  point P79 (-51.7871, -15.8225)
  point P80 (-50.7921, -18.2246)
  point P81 (-48.8021, -23.0287)
  point P82 (-55.4328, -22.961)
  point P83 (-49.7971, -20.6266)
  point P84 (-46.1034, -38.7495)
  point P85 (-41.79, -34.4361)
  point P86 (-39.9515, -36.2746)
  point P87 (-36.2746, -39.9515)
  point P88 (-42.4264, -42.4264)
  point P89 (-38.1131, -38.1131)
  point P90 (-27.7652, -53.4428)
  point P91 (-25.4308, -47.8072)
  point P92 (-23.0287, -48.8021)
  point P93 (-18.2246, -50.7921)
  point P94 (-22.961, -55.4328)
  point P95 (-20.6266, -49.7971)
  dimension "d89" = 360
  constraints: 800 end point, 6 parallel, 3 perpendicular, 2 coincident, 2 vertical, 1 vertical alignment, 928 other
sketch "Sketch5" plane through (0, 1, 0) normal (0, 1, 0) x (1, 0, 0)
  circle A0 centre (0, 0) radius 65
  line L0 (0, -65) -> (0, -63) construction
  line L1 (-3, -57) -> (-3, -63)
  line L2 (-3, -63) -> (3, -63)
  line L3 (3, -63) -> (3, -57)
  line L4 (3, -57) -> (-3, -57)
  line L5 (0.8, -52.3) -> (0.8, -55.5)
  line L6 (0.8, -55.5) -> (-0.8, -55.5)
  line L7 (-0.8, -55.5) -> (-0.8, -52.3)
  line L8 (-0.8, -52.3) -> (0.8, -52.3)
  line L9 (1.8, -52.3) -> (1.8, -55.5)
  line L10 (1.8, -55.5) -> (3.4, -55.5)
  line L11 (3.4, -55.5) -> (3.4, -52.3)
  line L12 (3.4, -52.3) -> (1.8, -52.3)
  line L13 (-1.8, -52.3) -> (-3.4, -52.3)
  line L14 (-3.4, -52.3) -> (-3.4, -55.5)
  line L15 (-3.4, -55.5) -> (-1.8, -55.5)
  line L16 (-1.8, -55.5) -> (-1.8, -52.3)
  line L17 (-4.4, -52.3) -> (-4.4, -55.5)
  line L18 (-6, -55.5) -> (-6, -52.3)
  line L19 (-6, -52.3) -> (-4.4, -52.3)
  line L20 (-4.4, -55.5) -> (-6, -55.5)
  line L21 (-4.4, -61.6) -> (-4.4, -58.4)
  line L22 (-4.4, -58.4) -> (-6, -58.4)
  line L23 (-6, -58.4) -> (-6, -61.6)
  line L24 (-6, -61.6) -> (-4.4, -61.6)
  line L25 (18.0977, -52.5764) -> (19.5759, -51.9641)
  line L26 (19.5759, -51.9641) -> (18.3514, -49.0077)
  line L27 (18.3514, -49.0077) -> (16.8732, -49.62)
  line L28 (16.8732, -49.62) -> (18.0977, -52.5764)
  line L29 (15.9493, -50.0027) -> (17.1739, -52.9591)
  line L30 (15.6957, -53.5714) -> (14.4711, -50.615)
  line L31 (14.4711, -50.615) -> (15.9493, -50.0027)
  line L32 (17.1739, -52.9591) -> (15.6957, -53.5714)
  line L33 (18.2836, -55.6384) -> (16.8054, -56.2507)
  line L34 (16.8054, -56.2507) -> (18.03, -59.2071)
  line L35 (18.03, -59.2071) -> (19.5082, -58.5948)
  line L36 (19.5082, -58.5948) -> (18.2836, -55.6384)
  line L37 (19.0413, -53.8092) -> (21.3374, -59.3525)
  line L38 (21.3374, -59.3525) -> (26.8807, -57.0564)
  line L39 (24.8744, -60.0522) -> (24.1091, -58.2044) construction
  line L40 (26.8807, -57.0564) -> (24.5846, -51.5131)
  line L41 (24.5846, -51.5131) -> (19.0413, -53.8092)
  line L42 (20.7534, -48.0128) -> (21.978, -50.9692)
  line L43 (21.978, -50.9692) -> (20.4998, -51.5815)
  line L44 (20.4998, -51.5815) -> (19.2752, -48.625)
  line L45 (19.2752, -48.625) -> (20.7534, -48.0128)
  line L46 (21.6773, -47.6301) -> (22.9019, -50.5865)
  line L47 (22.9019, -50.5865) -> (24.3801, -49.9742)
  line L48 (24.3801, -49.9742) -> (23.1555, -47.0178)
  line L49 (23.1555, -47.0178) -> (21.6773, -47.6301)
  line L50 (36.8403, -41.6486) -> (37.9716, -40.5172)
  line L51 (37.9716, -40.5172) -> (35.7089, -38.2545)
  line L52 (35.7089, -38.2545) -> (34.5775, -39.3858)
  line L53 (34.5775, -39.3858) -> (36.8403, -41.6486)
  line L54 (33.8704, -40.093) -> (36.1332, -42.3557)
  line L55 (35.0018, -43.4871) -> (32.739, -41.2243)
  line L56 (32.739, -41.2243) -> (33.8704, -40.093)
  line L57 (36.1332, -42.3557) -> (35.0018, -43.4871)
  line L58 (38.1838, -44.4063) -> (37.0524, -45.5377)
  line L59 (37.0524, -45.5377) -> (39.3151, -47.8004)
  line L60 (39.3151, -47.8004) -> (40.4465, -46.669)
  line L61 (40.4465, -46.669) -> (38.1838, -44.4063)
  line L62 (38.1838, -42.4264) -> (42.4264, -46.669)
  line L63 (42.4264, -46.669) -> (46.669, -42.4264)
  line L64 (45.9619, -45.9619) -> (44.5477, -44.5477) construction
  line L65 (46.669, -42.4264) -> (42.4264, -38.1838)
  line L66 (42.4264, -38.1838) -> (38.1838, -42.4264)
  line L67 (37.5474, -36.416) -> (39.8101, -38.6787)
  line L68 (39.8101, -38.6787) -> (38.6787, -39.8101)
  line L69 (38.6787, -39.8101) -> (36.416, -37.5474)
  line L70 (36.416, -37.5474) -> (37.5474, -36.416)
  line L71 (38.2545, -35.7089) -> (40.5172, -37.9716)
  line L72 (40.5172, -37.9716) -> (41.6486, -36.8403)
  line L73 (41.6486, -36.8403) -> (39.3858, -34.5775)
  line L74 (39.3858, -34.5775) -> (38.2545, -35.7089)
  line L75 (49.9742, -24.3801) -> (50.5865, -22.9019)
  line L76 (50.5865, -22.9019) -> (47.6301, -21.6773)
  line L77 (47.6301, -21.6773) -> (47.0178, -23.1555)
  line L78 (47.0178, -23.1555) -> (49.9742, -24.3801)
  line L79 (46.6351, -24.0794) -> (49.5915, -25.304)
  line L80 (48.9792, -26.7822) -> (46.0228, -25.5576)
  line L81 (46.0228, -25.5576) -> (46.6351, -24.0794)
  line L82 (49.5915, -25.304) -> (48.9792, -26.7822)
  line L83 (52.2708, -26.4138) -> (51.6585, -27.892)
  line L84 (51.6585, -27.892) -> (54.6149, -29.1166)
  line L85 (54.6149, -29.1166) -> (55.2272, -27.6384)
  line L86 (55.2272, -27.6384) -> (52.2708, -26.4138)
  line L87 (51.5131, -24.5846) -> (57.0564, -26.8807)
  line L88 (57.0564, -26.8807) -> (59.3525, -21.3374)
  line L89 (60.0522, -24.8744) -> (58.2044, -24.1091) construction
  line L90 (59.3525, -21.3374) -> (53.8092, -19.0413)
  line L91 (53.8092, -19.0413) -> (51.5131, -24.5846)
  line L92 (48.625, -19.2752) -> (51.5815, -20.4998)
  line L93 (51.5815, -20.4998) -> (50.9692, -21.978)
  line L94 (50.9692, -21.978) -> (48.0128, -20.7534)
  line L95 (48.0128, -20.7534) -> (48.625, -19.2752)
  line L96 (49.0077, -18.3514) -> (51.9641, -19.5759)
  line L97 (51.9641, -19.5759) -> (52.5764, -18.0977)
  line L98 (52.5764, -18.0977) -> (49.62, -16.8732)
  line L99 (49.62, -16.8732) -> (49.0077, -18.3514)
  line L100 (55.5, -3.4) -> (55.5, -1.8)
  line L101 (55.5, -1.8) -> (52.3, -1.8)
  line L102 (52.3, -1.8) -> (52.3, -3.4)
  line L103 (52.3, -3.4) -> (55.5, -3.4)
  line L104 (52.3, -4.4) -> (55.5, -4.4)
  line L105 (55.5, -6) -> (52.3, -6)
  line L106 (52.3, -6) -> (52.3, -4.4)
  line L107 (55.5, -4.4) -> (55.5, -6)
  line L108 (58.4, -4.4) -> (58.4, -6)
  line L109 (58.4, -6) -> (61.6, -6)
  line L110 (61.6, -6) -> (61.6, -4.4)
  line L111 (61.6, -4.4) -> (58.4, -4.4)
  line L112 (57, -3) -> (63, -3)
  line L113 (63, -3) -> (63, 3)
  line L114 (65, 0) -> (63, 0) construction
  line L115 (63, 3) -> (57, 3)
  line L116 (57, 3) -> (57, -3)
  line L117 (52.3, 0.8) -> (55.5, 0.8)
  line L118 (55.5, 0.8) -> (55.5, -0.8)
  line L119 (55.5, -0.8) -> (52.3, -0.8)
  line L120 (52.3, -0.8) -> (52.3, 0.8)
  line L121 (52.3, 1.8) -> (55.5, 1.8)
  line L122 (55.5, 1.8) -> (55.5, 3.4)
  line L123 (55.5, 3.4) -> (52.3, 3.4)
  line L124 (52.3, 3.4) -> (52.3, 1.8)
  point P0 (0, -53.9)
  point P1 (0, -60)
  point P2 (2.6, -53.9)
  point P3 (-2.6, -53.9)
  point P4 (-5.2, -53.9)
  point P5 (-5.2, -60)
  point P6 (18.1568, -57.4227)
  point P7 (15.8225, -51.7871)
  point P8 (18.2246, -50.7921)
  point P9 (23.0287, -48.8021)
  point P10 (22.961, -55.4328)
  point P11 (20.6266, -49.7971)
  point P12 (38.7495, -46.1034)
  point P13 (34.4361, -41.79)
  point P14 (36.2746, -39.9515)
  point P15 (39.9515, -36.2746)
  point P16 (42.4264, -42.4264)
  point P17 (38.1131, -38.1131)
  point P18 (53.4428, -27.7652)
  point P19 (47.8072, -25.4308)
  point P20 (48.8021, -23.0287)
  point P21 (50.7921, -18.2246)
  point P22 (55.4328, -22.961)
  point P23 (49.7971, -20.6266)
  point P24 (60, -5.2)
  point P25 (53.9, -5.2)
  point P26 (53.9, -2.6)
  point P27 (53.9, 2.6)
  point P28 (60, 0)
  point P29 (53.9, 0)
  point P30 (22.961, 0)
  point P31 (42.4264, 0)
  point P32 (55.5, 0)
  dimension "d94" = 90
  dimension "d95" = 60
  dimension "d96" = 53.9
  dimension "d97" = 2.6
  dimension "d98" = 5.2
  dimension "d99" = 2.6
  dimension "d100" = 5.2
  dimension "d111" = 22.961
  dimension "d112" = 42.4264
  dimension "d113" = 55.4328
  dimension "d114" = 22.961
  dimension "d115" = 42.4264
  dimension "d116" = 60
  dimension "d117" = 55.5
  constraints: 250 end point, 6 parallel, 3 perpendicular, 2 vertical, 1 coincident, 1 midpoint, 1 vertical alignment, 234 other
  measures "d95" distance of point (0, 0) point (0, -60)
  measures "d96" distance of point (0, 0) point (0, -53.9)
  measures "d97" distance of point (2.6, -53.9) point (0, -53.9)
  measures "d98" distance of point (-5.2, -53.9) point (0, -53.9)
  measures "d99" distance of point (-2.6, -53.9) point (0, -53.9)
  measures "d100" distance of point (-5.2, -60) point (0, -60)
  measures "d111" vertical distance of point (55.433, -22.961) point (55.5, 0)
  measures "d112" distance of point (42.426, 0) point (42.426, -42.426)
  measures "d113" distance of point (22.961, 0) point (22.961, -55.433)
  measures "d114" distance of point (22.961, 0) point (0, 0)
  measures "d115" distance of point (42.426, 0) point (0, 0)
  measures "d116" distance of point (60, 0) point (0, 0)
  measures "d117" distance from line of point (0, 0) L118
body "Solid2"
